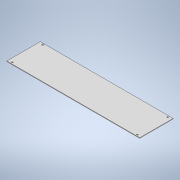
# Autodesk Inventor part: conveyor_backing_final
Saved by Autodesk Inventor 2022 (Build 260153000, 153)
## iProperties
Created: 2021-12-26
Part Number: conveyor_backing_final
Material: Generic
Document SubType Name: Modeling
Designer: Alex
Density: 1 g/cm^3
Appearance: Default
Author: Alex
Autodesk Inventor part; units mm, degrees
ref_plane "YZ Plane" through (0, 0, 0) normal (1, 0, 0) x (0, 1, 0)
ref_plane "XZ Plane" through (0, 0, 0) normal (0, 1, 0) x (-1, 0, 0)
ref_plane "XY Plane" through (0, 0, 0) normal (0, 0, 1) x (1, 0, 0)
sketch "Sketch1" plane through (0, 0, 0) normal (0, 1, 0) x (-1, 0, 0)
  line L0 (-431.8, -1.27) -> (-431.8, -109.982)
  line L1 (0, -109.982) -> (0, -1.27)
  circle A0 centre (-12.7, -6.35) radius 2.2225
  circle A1 centre (-12.7, -104.902) radius 2.2225
  circle A2 centre (-419.1, -6.35) radius 2.2225
  circle A3 centre (-419.1, -104.902) radius 2.2225
  line L2 (0, -109.982) -> (-431.8, -109.982)
  line L3 (0, -109.982) -> (431.8, -109.982) construction
  line L4 (0, -1.27) -> (-431.8, -1.27)
  point P0 (0, 0)
  dimension "d2" = 4.445
  dimension "d3" = 4.445
  dimension "d4" = 4.445
  dimension "d5" = 4.445
  dimension "d6" = 431.8
  constraints: 10 end point, 4 centre point, 1 collinear, 1 horizontal, 1 parallel, 1 perpendicular
  measures "d2" diameter of A0
  measures "d3" diameter of A1
  measures "d4" diameter of A2
  measures "d5" diameter of A3
  measures "d6" distance of L0.end L1.start
extrude "Extrusion1" add sketch "Sketch1" along normal blind 1.778
body "Solid1"
